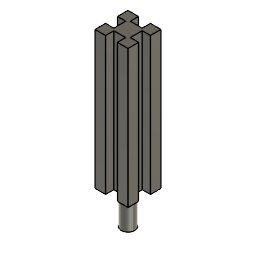
Pillar (Autodesk Fusion 360 design; units mm, degrees)
Autodesk Fusion 360 part; units mm, degrees
sketch "Sketch1" plane through (0, 0, 0) normal (0, 0, 1) x (1, 0, 0) in component "Pillar"
  line L0 (6, -6) -> (-6, -6)
  line L1 (-6, -6) -> (-6, 6)
  line L2 (-6, 6) -> (6, 6)
  line L3 (6, 6) -> (6, -6)
  line L4 (6, -6) -> (-6, 6) construction
  line L5 (-6, -6) -> (6, 6) construction
  dimension "d1" = 12
  dimension "d2" = 12
  constraint horizontal L0
  constraint perpendicular L0 L1
  constraint parallel L0 L2
  constraint parallel L1 L3
  constraint coincident L4 origin
  constraint coincident L5 origin
  measures "d1" distance of L1.end L2.end
  measures "d2" distance of L0.end L1.end
extrude "Extrude1" add sketch "Sketch1" along normal blind 50 in component "Pillar"
sketch "Sketch2" plane through (0, 0, 50) normal (0, 0, 1) x (-1, 0, 0) in component "Pillar"
  line L0 (-6, -6) -> (6, -6)
  line L1 (6, -6) -> (6, 6)
  line L2 (6, 6) -> (-6, 6)
  line L3 (-6, 6) -> (-6, -6)
  line L4 (-3, 2.15) -> (-9, 2.15)
  line L5 (-9, 2.15) -> (-9, -2.15)
  line L6 (-9, -2.15) -> (-3, -2.15)
  line L7 (-3, -2.15) -> (-3, 2.15)
  line L8 (-3, 2.15) -> (-9, -2.15) construction
  line L9 (-9, 2.15) -> (-3, -2.15) construction
  line L10 (2.15, -9) -> (-2.15, -9)
  line L11 (-2.15, -9) -> (-2.15, -3)
  line L12 (-2.15, -3) -> (2.15, -3)
  line L13 (2.15, -3) -> (2.15, -9)
  line L14 (2.15, -9) -> (-2.15, -3) construction
  line L15 (-2.15, -9) -> (2.15, -3) construction
  line L16 (9, -2.15) -> (3, -2.15)
  line L17 (3, -2.15) -> (3, 2.15)
  line L18 (3, 2.15) -> (9, 2.15)
  line L19 (9, 2.15) -> (9, -2.15)
  line L20 (9, -2.15) -> (3, 2.15) construction
  line L21 (3, -2.15) -> (9, 2.15) construction
  line L22 (-2.15, 9) -> (2.15, 9)
  line L23 (2.15, 9) -> (2.15, 3)
  line L24 (2.15, 3) -> (-2.15, 3)
  line L25 (-2.15, 3) -> (-2.15, 9)
  line L26 (-2.15, 9) -> (2.15, 3) construction
  line L27 (2.15, 9) -> (-2.15, 3) construction
  point P0 (-6, 0)
  point P1 (0, -6)
  point P2 (6, 0)
  point P3 (0, 6)
  dimension "d5" = 6
  dimension "d6" = 4.3
  dimension "d9" = 4.3
  dimension "d10" = 6
  dimension "d11" = 6
  dimension "d12" = 4.3
  dimension "d13" = 4.3
  dimension "d14" = 6
  constraint horizontal L4
  constraint perpendicular L4 L5
  constraint parallel L4 L6
  constraint parallel L5 L7
  constraint coincident L8 P0
  constraint coincident L9 P0
  constraint midpoint L3 P0
  constraint horizontal L10
  constraint perpendicular L10 L11
  constraint parallel L10 L12
  constraint parallel L11 L13
  constraint coincident L14 P1
  constraint coincident L15 P1
  constraint midpoint L0 P1
  constraint horizontal L16
  constraint perpendicular L16 L17
  constraint parallel L16 L18
  constraint parallel L17 L19
  constraint coincident L20 P2
  constraint coincident L21 P2
  constraint midpoint L1 P2
  constraint horizontal L22
  constraint perpendicular L22 L23
  constraint parallel L22 L24
  constraint parallel L23 L25
  constraint coincident L26 P3
  constraint coincident L27 P3
  constraint midpoint L2 P3
  measures "d5" distance of L5.end L6.end
  measures "d6" distance of L4.end L5.end
  measures "d9" distance of L11.end L12.end
  measures "d10" distance of L10.end L11.end
  measures "d11" distance of L17.end L18.end
  measures "d12" distance of L16.end L17.end
  measures "d13" distance of L23.end L24.end
  measures "d14" distance of L22.end L23.end
extrude "Extrude7" cut sketch "Sketch2" against normal blind 50 contours L0 L11 L12 L13 | L3 L4 L6 L7 | L1 L16 L17 L18 | L2 L23 L24 L25 in component "Pillar"
extrude "Extrude3" cut sketch "Sketch2" against normal blind 30 contours L0 L11 L12 L13 in component "Pillar"
extrude "Extrude2" cut sketch "Sketch2" against normal blind 30 contours L3 L4 L6 L7 in component "Pillar"
extrude "Extrude4" cut sketch "Sketch2" against normal blind 30 contours L1 L16 L17 L18 in component "Pillar"
extrude "Extrude5" cut sketch "Sketch2" against normal blind 30 contours L2 L23 L24 L25 in component "Pillar"
sketch "Sketch3" plane through (0, 0, 0) normal (0, 0, -1) x (1, 0, 0) in component "Pillar"
  line L0 (2.15, -6) -> (6, -6)
  line L1 (6, -6) -> (6, -2.15)
  line L2 (6, 6) -> (2.15, 6)
  line L3 (-6, 6) -> (-6, 2.15)
  circle A0 centre (0, 0) radius 2.5
  line L4 (-2.15, -6) -> (-2.15, -3)
  line L5 (-2.15, -3) -> (2.15, -3)
  line L6 (2.15, -3) -> (2.15, -6)
  line L7 (6, -2.15) -> (3, -2.15)
  line L8 (3, -2.15) -> (3, 2.15)
  line L9 (3, 2.15) -> (6, 2.15)
  line L10 (6, 2.15) -> (6, 6)
  line L11 (2.15, 6) -> (2.15, 3)
  line L12 (2.15, 3) -> (-2.15, 3)
  line L13 (-2.15, 3) -> (-2.15, 6)
  line L14 (-2.15, 6) -> (-6, 6)
  line L15 (-6, 2.15) -> (-3, 2.15)
  line L16 (-3, 2.15) -> (-3, -2.15)
  line L17 (-3, -2.15) -> (-6, -2.15)
  line L18 (-6, -2.15) -> (-6, -6)
  line L19 (-6, -6) -> (-2.15, -6)
  dimension "d21" = 5
  constraint coincident A0.centre origin
  measures "d21" diameter of A0
extrude "Extrude6" add sketch "Sketch3" along normal blind 12 contours A0 in component "Pillar"
component "Pillar" placed x (1, 0, 0) y (0, 1, 0) z (0, 0, 1) at (0, 0, 0)
